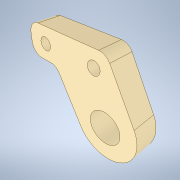
# Autodesk Inventor part: Рычаг фиксатора 2
Saved by Autodesk Inventor 2021.1 (Build 251245010, 245A)
## iProperties
Created: 2026-04-13
Part Number: Рычаг фиксатора 2
Material: Типовые
Document SubType Name: Modeling
Designer: Андрей Тарасов
Density: 1 g/cm^3
Appearance: По умолчанию
Author: Андрей Тарасов
Autodesk Inventor part; units mm, degrees
ref_plane "YZ Plane" through (0, 0, 0) normal (1, 0, 0) x (0, 1, 0)
ref_plane "XZ Plane" through (0, 0, 0) normal (0, 1, 0) x (-1, 0, 0)
ref_plane "XY Plane" through (0, 0, 0) normal (0, 0, 1) x (1, 0, 0)
sketch "Эскиз1" plane through (0, 0, 0) normal (0, 0, 1) x (1, 0, 0)
  circle A0 centre (0, 0) radius 5.1
  circle A1 centre (66, 0) radius 4
  line L0 (-20.92, 0) -> (89.82, 0) construction
  line L1 (-5.1, 0) -> (-5.1, 14) construction
  line L2 (5.1, 0) -> (5.1, 14) construction
  line L3 (-4.85, 1.5772) -> (-4.85, 16.5)
  line L4 (-4.85, 16.5) -> (65.7113, 16.5)
  line L5 (65.7113, 16.5) -> (72.9282, 4)
  line L6 (59.0718, -4) -> (51.8549, 8.5)
  line L7 (4.85, 16.5) -> (4.85, 1.5772)
  line L8 (4.85, 8.5) -> (70.3301, 8.5)
  circle A2 centre (66, 0) radius 8
  line L9 (51.8549, 8.5) -> (51.8549, 16.5) construction
  line L10 (68.0207, 12.5) -> (-4.85, 12.5) construction
  circle A3 centre (62.8549, 12.5) radius 1.6
  circle A4 centre (15.15, 12.5) radius 1.6
  circle A5 centre (48.8549, 12.5) radius 1.6
  line L11 (43.8549, 8.5) -> (43.8549, 16.5)
  point P0 (43.8549, 12.5)
  dimension "d0" = 10.2
  dimension "d1" = 8
  dimension "d2" = 66
  dimension "d3" = 0.25
  dimension "d4" = 0.25
  dimension "d5" = 8.5
  dimension "d6" = 16
  dimension "d7" = 60
  dimension "d8" = 8
  dimension "d9" = 3.2
  dimension "d10" = 3.2
  dimension "d12" = 20
  dimension "d18" = 3.2
  dimension "d20" = 14
  dimension "d21" = 8
  dimension "d22" = 5
  constraints: 22 end point, 16 point on line, 6 centre point, 6 perpendicular, 6 point on circle, 4 tangent, 2 coincident, 2 parallel, 1 horizontal, 1 midpoint
  measures "d0" diameter of A0
  measures "d1" diameter of A1
  measures "d2" distance of A1.centre point (0, 0)
  measures "d3" distance between parallel lines of L3 L1
  measures "d4" distance between parallel lines of L2 L7
  measures "d5" distance between parallel lines of L8 L0
  measures "d6" diameter of A2
  measures "d7" angle of L0 L6
  measures "d8" distance between parallel lines of L4 L8
  measures "d9" diameter of A3
  measures "d10" diameter of A4
  measures "d12" distance from line of L3 A4.centre
  measures "d18" diameter of A5
  measures "d20" distance of A5.centre A3.centre
  measures "d21" distance between parallel lines of L9 L11
  measures "d22" distance from line of A5.centre L11
extrude "Выдавливание1" add sketch "Эскиз1" along normal blind 6 contours L11 L4 L5 L8 | L8 L5 A2 L6 | A2
fillet "Сопряжение1" radius 3 4 edges at (51.8549, 8.5, 3) (65.7113, 16.5, 3) (43.8549, 16.5, 3) (43.8549, 8.5, 3)
equation "\"d4\" = d3"
equation "\"d10\" = d18"
equation "\"d18\" = d9"
